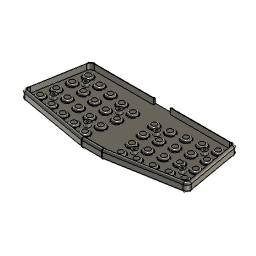
pusheenz40 low tolerance v5 (Autodesk Fusion 360 design; units mm, degrees)
Autodesk Fusion 360 part; units mm, degrees
note: some values were not read from the file. Chosen so that the rebuilt part matches the saved one: which bodies a step acts on. Set by a fixed rule: which sketch regions a step uses.
(part 1 of 2)
sketch "Sketch1" plane through (0, 0, 0) normal (0, 0, 1) x (1, 0, 0)
  line L0 (-7.5882, -2.7237) -> (-0.9058, 35.1744)
  line L1 (2.0486, 37.6534) -> (102.6819, 37.6534)
  line L2 (105.6363, 35.1744) -> (112.3188, -2.7237)
  line L3 (109.8853, -6.1991) -> (59.9186, -15.0095)
  line L4 (59.3977, -15.0551) -> (45.3329, -15.0551)
  line L5 (44.8119, -15.0095) -> (-5.1548, -6.1991)
  arc A0 (2.0486, 37.6534) -> (-0.9058, 35.1744) centre (2.0486, 34.6534) ccw
  arc A1 (105.6363, 35.1744) -> (102.6819, 37.6534) centre (102.6819, 34.6534) ccw
  arc A2 (109.8853, -6.1991) -> (112.3188, -2.7237) centre (109.3644, -3.2446) ccw
  arc A3 (59.3977, -15.0551) -> (59.9186, -15.0095) centre (59.3977, -12.0551) ccw
  arc A4 (44.8119, -15.0095) -> (45.3329, -15.0551) centre (45.3329, -12.0551) ccw
  arc A5 (-7.5882, -2.7237) -> (-5.1548, -6.1991) centre (-4.6338, -3.2446) ccw
  line L6 (-5.8506, -1.507) -> (0.3109, 33.4367)
  line L7 (3.2654, 35.9157) -> (101.4652, 35.9157)
  line L8 (104.4196, 33.4367) -> (110.5811, -1.507)
  line L9 (108.1476, -4.9823) -> (61.1353, -13.2719)
  line L10 (60.6144, -13.3174) -> (44.1162, -13.3174)
  line L11 (43.5952, -13.2719) -> (-3.4171, -4.9823)
  arc A6 (3.2654, 35.9157) -> (0.3109, 33.4367) centre (3.2654, 32.9157) ccw
  arc A7 (104.4196, 33.4367) -> (101.4652, 35.9157) centre (101.4652, 32.9157) ccw
  arc A8 (108.1476, -4.9823) -> (110.5811, -1.507) centre (107.6267, -2.0279) ccw
  arc A9 (60.6144, -13.3174) -> (61.1353, -13.2719) centre (60.6144, -10.3174) ccw
  arc A10 (43.5952, -13.2719) -> (44.1162, -13.3174) centre (44.1162, -10.3174) ccw
  arc A11 (-5.8506, -1.507) -> (-3.4171, -4.9823) centre (-2.8961, -2.0279) ccw
  line L12 (-5.2713, -1.1014) -> (0.7165, 32.8575)
  line L13 (3.6709, 35.3365) -> (101.0596, 35.3365)
  line L14 (104.014, 32.8575) -> (110.0019, -1.1014)
  line L15 (107.5684, -4.5767) -> (61.5409, -12.6926)
  line L16 (61.02, -12.7382) -> (43.7106, -12.7382)
  line L17 (43.1896, -12.6926) -> (-2.8379, -4.5767)
  arc A12 (3.6709, 35.3365) -> (0.7165, 32.8575) centre (3.6709, 32.3365) ccw
  arc A13 (104.014, 32.8575) -> (101.0596, 35.3365) centre (101.0596, 32.3365) ccw
  arc A14 (107.5684, -4.5767) -> (110.0019, -1.1014) centre (107.0475, -1.6223) ccw
  arc A15 (61.02, -12.7382) -> (61.5409, -12.6926) centre (61.02, -9.7382) ccw
  arc A16 (43.1896, -12.6926) -> (43.7106, -12.7382) centre (43.7106, -9.7382) ccw
  arc A17 (-5.2713, -1.1014) -> (-2.8379, -4.5767) centre (-2.3169, -1.6223) ccw
  arc A18 (-3.5838, -0.4343) -> (3.2191, -1.6338) centre (0, 0) ccw
  arc A19 (3.5838, 0.4343) -> (-3.2191, 1.6338) centre (0, 0) ccw
  arc A20 (-1.8473, 9.4138) -> (4.9556, 8.2143) centre (1.7365, 9.8481) ccw
  arc A21 (5.3203, 10.2824) -> (-1.4826, 11.4819) centre (1.7365, 9.8481) ccw
  arc A22 (-0.1108, 19.2619) -> (6.6921, 18.0623) centre (3.473, 19.6962) ccw
  arc A23 (7.0567, 20.1304) -> (0.2538, 21.33) centre (3.473, 19.6962) ccw
  arc A24 (1.6257, 29.11) -> (8.4286, 27.9104) centre (5.2094, 29.5442) ccw
  arc A25 (8.7932, 29.9785) -> (1.9903, 31.178) centre (5.2094, 29.5442) ccw
  arc A26 (6.2643, -2.1708) -> (13.0672, -3.3703) centre (9.8481, -1.7365) ccw
  arc A27 (13.4319, -1.3022) -> (6.629, -0.1027) centre (9.8481, -1.7365) ccw
  arc A28 (8.0008, 7.6773) -> (14.8037, 6.4778) centre (11.5846, 8.1116) ccw
  arc A29 (15.1683, 8.5459) -> (8.3654, 9.7454) centre (11.5846, 8.1116) ccw
  arc A30 (9.7373, 17.5254) -> (16.5402, 16.3259) centre (13.321, 17.9597) ccw
  arc A31 (16.9048, 18.394) -> (10.1019, 19.5935) centre (13.321, 17.9597) ccw
  arc A32 (11.4737, 27.3735) -> (18.2766, 26.1739) centre (15.0575, 27.8078) ccw
  arc A33 (18.6413, 28.242) -> (11.8384, 29.4416) centre (15.0575, 27.8078) ccw
  arc A34 (16.1124, -3.9072) -> (22.9153, -5.1068) centre (19.6962, -3.473) ccw
  arc A35 (23.2799, -3.0387) -> (16.477, -1.8391) centre (19.6962, -3.473) ccw
  arc A36 (17.8489, 5.9408) -> (24.6518, 4.7413) centre (21.4326, 6.3751) ccw
  arc A37 (25.0164, 6.8094) -> (18.2135, 8.0089) centre (21.4326, 6.3751) ccw
  arc A38 (19.5853, 15.7889) -> (26.3882, 14.5894) centre (23.1691, 16.2232) ccw
  arc A39 (26.7529, 16.6575) -> (19.95, 17.857) centre (23.1691, 16.2232) ccw
  arc A40 (21.3218, 25.637) -> (28.1247, 24.4375) centre (24.9056, 26.0713) ccw
  arc A41 (28.4894, 26.5055) -> (21.6865, 27.7051) centre (24.9056, 26.0713) ccw
  arc A42 (25.9604, -5.6437) -> (32.7634, -6.8433) centre (29.5442, -5.2094) ccw
  arc A43 (33.128, -4.7752) -> (26.3251, -3.5756) centre (29.5442, -5.2094) ccw
  arc A44 (27.6969, 4.2044) -> (34.4998, 3.0048) centre (31.2807, 4.6386) ccw
  arc A45 (34.8645, 5.0729) -> (28.0616, 6.2724) centre (31.2807, 4.6386) ccw
  arc A46 (29.4334, 14.0524) -> (36.2363, 12.8529) centre (33.0172, 14.4867) ccw
  arc A47 (36.601, 14.921) -> (29.7981, 16.1205) centre (33.0172, 14.4867) ccw
  arc A48 (31.1699, 23.9005) -> (37.9728, 22.701) centre (34.7537, 24.3348) ccw
  arc A49 (38.3375, 24.7691) -> (31.5346, 25.9686) centre (34.7537, 24.3348) ccw
  arc A50 (35.8085, -7.3802) -> (42.6114, -8.5797) centre (39.3923, -6.9459) ccw
  arc A51 (42.9761, -6.5116) -> (36.1732, -5.3121) centre (39.3923, -6.9459) ccw
  arc A52 (37.545, 2.4679) -> (44.3479, 1.2683) centre (41.1288, 2.9022) ccw
  arc A53 (44.7126, 3.3364) -> (37.9097, 4.536) centre (41.1288, 2.9022) ccw
  arc A54 (39.2815, 12.3159) -> (46.0844, 11.1164) centre (42.8653, 12.7502) ccw
  arc A55 (46.4491, 13.1845) -> (39.6462, 14.384) centre (42.8653, 12.7502) ccw
  arc A56 (41.018, 22.164) -> (47.8209, 20.9645) centre (44.6018, 22.5983) ccw
  arc A57 (48.1855, 23.0326) -> (41.3826, 24.2321) centre (44.6018, 22.5983) ccw
  arc A58 (101.5114, -1.6338) -> (108.3143, -0.4343) centre (104.7305, 0) ccw
  arc A59 (107.9497, 1.6338) -> (101.1468, 0.4343) centre (104.7305, 0) ccw
  arc A60 (99.7749, 8.2143) -> (106.5778, 9.4138) centre (102.9941, 9.8481) ccw
  arc A61 (106.2132, 11.4819) -> (99.4103, 10.2824) centre (102.9941, 9.8481) ccw
  arc A62 (98.0385, 18.0623) -> (104.8414, 19.2619) centre (101.2576, 19.6962) ccw
  arc A63 (104.4767, 21.33) -> (97.6738, 20.1304) centre (101.2576, 19.6962) ccw
  arc A64 (96.302, 27.9104) -> (103.1049, 29.11) centre (99.5211, 29.5442) ccw
  arc A65 (102.7402, 31.178) -> (95.9373, 29.9785) centre (99.5211, 29.5442) ccw
  arc A66 (91.6633, -3.3703) -> (98.4663, -2.1708) centre (94.8825, -1.7365) ccw
  arc A67 (98.1016, -0.1027) -> (91.2987, -1.3022) centre (94.8825, -1.7365) ccw
  arc A68 (89.9269, 6.4778) -> (96.7298, 7.6773) centre (93.146, 8.1116) ccw
  arc A69 (96.3651, 9.7454) -> (89.5622, 8.5459) centre (93.146, 8.1116) ccw
  arc A70 (88.1904, 16.3259) -> (94.9933, 17.5254) centre (91.4095, 17.9597) ccw
  arc A71 (94.6286, 19.5935) -> (87.8257, 18.394) centre (91.4095, 17.9597) ccw
  arc A72 (86.4539, 26.1739) -> (93.2568, 27.3735) centre (89.673, 27.8078) ccw
  arc A73 (92.8921, 29.4416) -> (86.0892, 28.242) centre (89.673, 27.8078) ccw
  arc A74 (81.8153, -5.1068) -> (88.6182, -3.9072) centre (85.0344, -3.473) ccw
  arc A75 (88.2535, -1.8391) -> (81.4506, -3.0387) centre (85.0344, -3.473) ccw
  arc A76 (80.0788, 4.7413) -> (86.8817, 5.9408) centre (83.2979, 6.3751) ccw
  arc A77 (86.517, 8.0089) -> (79.7141, 6.8094) centre (83.2979, 6.3751) ccw
  arc A78 (78.3423, 14.5894) -> (85.1452, 15.7889) centre (81.5614, 16.2232) ccw
  arc A79 (84.7806, 17.857) -> (77.9776, 16.6575) centre (81.5614, 16.2232) ccw
  arc A80 (76.6058, 24.4375) -> (83.4087, 25.637) centre (79.8249, 26.0713) ccw
  arc A81 (83.0441, 27.7051) -> (76.2412, 26.5055) centre (79.8249, 26.0713) ccw
  arc A82 (71.9672, -6.8433) -> (78.7701, -5.6437) centre (75.1863, -5.2094) ccw
  arc A83 (78.4054, -3.5756) -> (71.6025, -4.7752) centre (75.1863, -5.2094) ccw
  arc A84 (70.2307, 3.0048) -> (77.0336, 4.2044) centre (73.4498, 4.6386) ccw
  arc A85 (76.669, 6.2724) -> (69.866, 5.0729) centre (73.4498, 4.6386) ccw
  arc A86 (68.4942, 12.8529) -> (75.2971, 14.0524) centre (71.7134, 14.4867) ccw
  arc A87 (74.9325, 16.1205) -> (68.1296, 14.921) centre (71.7134, 14.4867) ccw
  arc A88 (66.7577, 22.701) -> (73.5607, 23.9005) centre (69.9769, 24.3348) ccw
  arc A89 (73.196, 25.9686) -> (66.3931, 24.7691) centre (69.9769, 24.3348) ccw
  arc A90 (62.1191, -8.5797) -> (68.922, -7.3802) centre (65.3382, -6.9459) ccw
  arc A91 (68.5574, -5.3121) -> (61.7545, -6.5116) centre (65.3382, -6.9459) ccw
  arc A92 (60.3826, 1.2683) -> (67.1855, 2.4679) centre (63.6018, 2.9022) ccw
  arc A93 (66.8209, 4.536) -> (60.018, 3.3364) centre (63.6018, 2.9022) ccw
  arc A94 (58.6462, 11.1164) -> (65.4491, 12.3159) centre (61.8653, 12.7502) ccw
  arc A95 (65.0844, 14.384) -> (58.2815, 13.1845) centre (61.8653, 12.7502) ccw
  arc A96 (56.9097, 20.9645) -> (63.7126, 22.164) centre (60.1288, 22.5983) ccw
  arc A97 (63.3479, 24.2321) -> (56.545, 23.0326) centre (60.1288, 22.5983) ccw
  line L18 (-3.5838, -0.4343) -> (-3.0862, -0.522)
  line L19 (2.7215, -1.5461) -> (3.2191, -1.6338)
  line L20 (3.5838, 0.4343) -> (3.0862, 0.522)
  line L21 (-2.7215, 1.5461) -> (-3.2191, 1.6338)
  line L22 (-1.8473, 9.4138) -> (-1.3497, 9.3261)
  line L23 (4.458, 8.302) -> (4.9556, 8.2143)
  line L24 (5.3203, 10.2824) -> (4.8226, 10.3701)
  line L25 (-0.985, 11.3941) -> (-1.4826, 11.4819)
  line L26 (-0.1108, 19.2619) -> (0.3868, 19.1741)
  line L27 (6.1945, 18.1501) -> (6.6921, 18.0623)
  line L28 (7.0567, 20.1304) -> (6.5591, 20.2182)
  line L29 (0.7515, 21.2422) -> (0.2538, 21.33)
  line L30 (1.6257, 29.11) -> (2.1233, 29.0222)
  line L31 (7.9309, 27.9982) -> (8.4286, 27.9104)
  line L32 (8.7932, 29.9785) -> (8.2956, 30.0663)
  line L33 (2.4879, 31.0903) -> (1.9903, 31.178)
  line L34 (6.2643, -2.1708) -> (6.7619, -2.2585)
  line L35 (12.5696, -3.2826) -> (13.0672, -3.3703)
  line L36 (13.4319, -1.3022) -> (12.9342, -1.2145)
  line L37 (7.1266, -0.1904) -> (6.629, -0.1027)
  line L38 (8.0008, 7.6773) -> (8.4984, 7.5896)
  line L39 (14.3061, 6.5655) -> (14.8037, 6.4778)
  line L40 (15.1683, 8.5459) -> (14.6707, 8.6336)
  line L41 (8.8631, 9.6577) -> (8.3654, 9.7454)
  line L42 (9.7373, 17.5254) -> (10.2349, 17.4376)
  line L43 (16.0425, 16.4136) -> (16.5402, 16.3259)
  line L44 (16.9048, 18.394) -> (16.4072, 18.4817)
  line L45 (10.5995, 19.5057) -> (10.1019, 19.5935)
  line L46 (11.4737, 27.3735) -> (11.9714, 27.2857)
  line L47 (17.779, 26.2617) -> (18.2766, 26.1739)
  line L48 (18.6413, 28.242) -> (18.1437, 28.3298)
  line L49 (12.336, 29.3538) -> (11.8384, 29.4416)
  line L50 (16.1124, -3.9072) -> (16.61, -3.995)
  line L51 (22.4177, -5.019) -> (22.9153, -5.1068)
  line L52 (23.2799, -3.0387) -> (22.7823, -2.9509)
  line L53 (16.9747, -1.9269) -> (16.477, -1.8391)
  line L54 (17.8489, 5.9408) -> (18.3465, 5.8531)
  line L55 (24.1541, 4.829) -> (24.6518, 4.7413)
  line L56 (25.0164, 6.8094) -> (24.5188, 6.8971)
  line L57 (18.7111, 7.9212) -> (18.2135, 8.0089)
  line L58 (19.5853, 15.7889) -> (20.083, 15.7012)
  line L59 (25.8906, 14.6771) -> (26.3882, 14.5894)
  line L60 (26.7529, 16.6575) -> (26.2553, 16.7452)
  line L61 (20.4476, 17.7693) -> (19.95, 17.857)
  line L62 (21.3218, 25.637) -> (21.8194, 25.5492)
  line L63 (27.6271, 24.5252) -> (28.1247, 24.4375)
  line L64 (28.4894, 26.5055) -> (27.9918, 26.5933)
  line L65 (22.1841, 27.6173) -> (21.6865, 27.7051)
  line L66 (25.9604, -5.6437) -> (26.4581, -5.7315)
  line L67 (32.2657, -6.7555) -> (32.7634, -6.8433)
  line L68 (33.128, -4.7752) -> (32.6304, -4.6874)
  line L69 (26.8227, -3.6634) -> (26.3251, -3.5756)
  line L70 (27.6969, 4.2044) -> (28.1946, 4.1166)
  line L71 (34.0022, 3.0926) -> (34.4998, 3.0048)
  line L72 (34.8645, 5.0729) -> (34.3669, 5.1607)
  line L73 (28.5592, 6.1847) -> (28.0616, 6.2724)
  line L74 (29.4334, 14.0524) -> (29.931, 13.9647)
  line L75 (35.7387, 12.9406) -> (36.2363, 12.8529)
  line L76 (36.601, 14.921) -> (36.1034, 15.0087)
  line L77 (30.2957, 16.0328) -> (29.7981, 16.1205)
  line L78 (31.1699, 23.9005) -> (31.6675, 23.8128)
  line L79 (37.4752, 22.7887) -> (37.9728, 22.701)
  line L80 (38.3375, 24.7691) -> (37.8398, 24.8568)
  line L81 (32.0322, 25.8809) -> (31.5346, 25.9686)
  line L82 (35.8085, -7.3802) -> (36.3061, -7.468)
  line L83 (42.1138, -8.492) -> (42.6114, -8.5797)
  line L84 (42.9761, -6.5116) -> (42.4785, -6.4239)
  line L85 (36.6708, -5.3999) -> (36.1732, -5.3121)
  line L86 (37.545, 2.4679) -> (38.0426, 2.3801)
  line L87 (43.8503, 1.3561) -> (44.3479, 1.2683)
  line L88 (44.7126, 3.3364) -> (44.215, 3.4242)
  line L89 (38.4073, 4.4482) -> (37.9097, 4.536)
  line L90 (39.2815, 12.3159) -> (39.7791, 12.2282)
  line L91 (45.5868, 11.2042) -> (46.0844, 11.1164)
  line L92 (46.4491, 13.1845) -> (45.9514, 13.2723)
  line L93 (40.1438, 14.2963) -> (39.6462, 14.384)
  line L94 (41.018, 22.164) -> (41.5156, 22.0763)
  line L95 (47.3233, 21.0522) -> (47.8209, 20.9645)
  line L96 (48.1855, 23.0326) -> (47.6879, 23.1203)
  line L97 (41.8803, 24.1444) -> (41.3826, 24.2321)
  line L98 (101.5114, -1.6338) -> (102.009, -1.5461)
  line L99 (107.8167, -0.522) -> (108.3143, -0.4343)
  line L100 (107.9497, 1.6338) -> (107.452, 1.5461)
  line L101 (101.6444, 0.522) -> (101.1468, 0.4343)
  line L102 (99.7749, 8.2143) -> (100.2726, 8.302)
  line L103 (106.0802, 9.3261) -> (106.5778, 9.4138)
  line L104 (106.2132, 11.4819) -> (105.7156, 11.3941)
  line L105 (99.9079, 10.3701) -> (99.4103, 10.2824)
  line L106 (98.0385, 18.0623) -> (98.5361, 18.1501)
  line L107 (104.3437, 19.1741) -> (104.8414, 19.2619)
  line L108 (104.4767, 21.33) -> (103.9791, 21.2422)
  line L109 (98.1714, 20.2182) -> (97.6738, 20.1304)
  line L110 (96.302, 27.9104) -> (96.7996, 27.9982)
  line L111 (102.6073, 29.0222) -> (103.1049, 29.11)
  line L112 (102.7402, 31.178) -> (102.2426, 31.0903)
  line L113 (96.4349, 30.0663) -> (95.9373, 29.9785)
  line L114 (91.6633, -3.3703) -> (92.161, -3.2826)
  line L115 (97.9686, -2.2585) -> (98.4663, -2.1708)
  line L116 (98.1016, -0.1027) -> (97.604, -0.1904)
  line L117 (91.7963, -1.2145) -> (91.2987, -1.3022)
  line L118 (89.9269, 6.4778) -> (90.4245, 6.5655)
  line L119 (96.2321, 7.5896) -> (96.7298, 7.6773)
  line L120 (96.3651, 9.7454) -> (95.8675, 9.6577)
  line L121 (90.0598, 8.6336) -> (89.5622, 8.5459)
  line L122 (88.1904, 16.3259) -> (88.688, 16.4136)
  line L123 (94.4957, 17.4376) -> (94.9933, 17.5254)
  line L124 (94.6286, 19.5935) -> (94.131, 19.5057)
  line L125 (88.3233, 18.4817) -> (87.8257, 18.394)
  line L126 (86.4539, 26.1739) -> (86.9515, 26.2617)
  line L127 (92.7592, 27.2857) -> (93.2568, 27.3735)
  line L128 (92.8921, 29.4416) -> (92.3945, 29.3538)
  line L129 (86.5869, 28.3298) -> (86.0892, 28.242)
  line L130 (81.8153, -5.1068) -> (82.3129, -5.019)
  line L131 (88.1206, -3.995) -> (88.6182, -3.9072)
  line L132 (88.2535, -1.8391) -> (87.7559, -1.9269)
  line L133 (81.9482, -2.9509) -> (81.4506, -3.0387)
  line L134 (80.0788, 4.7413) -> (80.5764, 4.829)
  line L135 (86.3841, 5.8531) -> (86.8817, 5.9408)
  line L136 (86.517, 8.0089) -> (86.0194, 7.9212)
  line L137 (80.2117, 6.8971) -> (79.7141, 6.8094)
  line L138 (78.3423, 14.5894) -> (78.8399, 14.6771)
  line L139 (84.6476, 15.7012) -> (85.1452, 15.7889)
  line L140 (84.7806, 17.857) -> (84.2829, 17.7693)
  line L141 (78.4753, 16.7452) -> (77.9776, 16.6575)
  line L142 (76.6058, 24.4375) -> (77.1034, 24.5252)
  line L143 (82.9111, 25.5492) -> (83.4087, 25.637)
  line L144 (83.0441, 27.7051) -> (82.5464, 27.6173)
  line L145 (76.7388, 26.5933) -> (76.2412, 26.5055)
  line L146 (71.9672, -6.8433) -> (72.4648, -6.7555)
  line L147 (78.2725, -5.7315) -> (78.7701, -5.6437)
  line L148 (78.4054, -3.5756) -> (77.9078, -3.6634)
  line L149 (72.1002, -4.6874) -> (71.6025, -4.7752)
  line L150 (70.2307, 3.0048) -> (70.7283, 3.0926)
  line L151 (76.536, 4.1166) -> (77.0336, 4.2044)
  line L152 (76.669, 6.2724) -> (76.1713, 6.1847)
  line L153 (70.3637, 5.1607) -> (69.866, 5.0729)
  line L154 (68.4942, 12.8529) -> (68.9919, 12.9406)
  line L155 (74.7995, 13.9647) -> (75.2971, 14.0524)
  line L156 (74.9325, 16.1205) -> (74.4349, 16.0328)
  line L157 (68.6272, 15.0087) -> (68.1296, 14.921)
  line L158 (66.7577, 22.701) -> (67.2554, 22.7887)
  line L159 (73.063, 23.8128) -> (73.5607, 23.9005)
  line L160 (73.196, 25.9686) -> (72.6984, 25.8809)
  line L161 (66.8907, 24.8568) -> (66.3931, 24.7691)
  line L162 (62.1191, -8.5797) -> (62.6167, -8.492)
  line L163 (68.4244, -7.468) -> (68.922, -7.3802)
  line L164 (68.5574, -5.3121) -> (68.0597, -5.3999)
  line L165 (62.2521, -6.4239) -> (61.7545, -6.5116)
  line L166 (60.3826, 1.2683) -> (60.8803, 1.3561)
  line L167 (66.6879, 2.3801) -> (67.1855, 2.4679)
  line L168 (66.8209, 4.536) -> (66.3233, 4.4482)
  line L169 (60.5156, 3.4242) -> (60.018, 3.3364)
  line L170 (58.6462, 11.1164) -> (59.1438, 11.2042)
  line L171 (64.9514, 12.2282) -> (65.4491, 12.3159)
  line L172 (65.0844, 14.384) -> (64.5868, 14.2963)
  line L173 (58.7791, 13.2723) -> (58.2815, 13.1845)
  line L174 (56.9097, 20.9645) -> (57.4073, 21.0522)
  line L175 (63.215, 22.0763) -> (63.7126, 22.164)
  line L176 (63.3479, 24.2321) -> (62.8503, 24.1444)
  line L177 (57.0426, 23.1203) -> (56.545, 23.0326)
  arc A98 (-3.0862, -0.522) -> (-3.0862, -0.522) centre (0, 0) ccw
  arc A99 (-1.3497, 9.3261) -> (-1.3497, 9.3261) centre (1.7365, 9.8481) ccw
  arc A100 (0.3868, 19.1741) -> (0.3868, 19.1741) centre (3.473, 19.6962) ccw
  arc A101 (2.1233, 29.0222) -> (2.1233, 29.0222) centre (5.2094, 29.5442) ccw
  arc A102 (6.7619, -2.2585) -> (6.7619, -2.2585) centre (9.8481, -1.7365) ccw
  arc A103 (8.4984, 7.5896) -> (8.4984, 7.5896) centre (11.5846, 8.1116) ccw
  arc A104 (10.2349, 17.4376) -> (10.2349, 17.4376) centre (13.321, 17.9597) ccw
  arc A105 (11.9714, 27.2857) -> (11.9714, 27.2857) centre (15.0575, 27.8078) ccw
  arc A106 (16.61, -3.995) -> (16.61, -3.995) centre (19.6962, -3.473) ccw
  arc A107 (18.3465, 5.8531) -> (18.3465, 5.8531) centre (21.4326, 6.3751) ccw
  arc A108 (20.083, 15.7012) -> (20.083, 15.7012) centre (23.1691, 16.2232) ccw
  arc A109 (21.8194, 25.5492) -> (21.8194, 25.5492) centre (24.9056, 26.0713) ccw
  arc A110 (26.4581, -5.7315) -> (26.4581, -5.7315) centre (29.5442, -5.2094) ccw
  arc A111 (28.1946, 4.1166) -> (28.1946, 4.1166) centre (31.2807, 4.6386) ccw
  arc A112 (29.931, 13.9647) -> (29.931, 13.9647) centre (33.0172, 14.4867) ccw
  arc A113 (31.6675, 23.8128) -> (31.6675, 23.8128) centre (34.7537, 24.3348) ccw
  arc A114 (36.3061, -7.468) -> (36.3061, -7.468) centre (39.3923, -6.9459) ccw
  arc A115 (38.0426, 2.3801) -> (38.0426, 2.3801) centre (41.1288, 2.9022) ccw
  arc A116 (39.7791, 12.2282) -> (39.7791, 12.2282) centre (42.8653, 12.7502) ccw
  arc A117 (41.5156, 22.0763) -> (41.5156, 22.0763) centre (44.6018, 22.5983) ccw
  arc A118 (102.009, -1.5461) -> (102.009, -1.5461) centre (104.7305, 0) ccw
  arc A119 (100.2726, 8.302) -> (100.2726, 8.302) centre (102.9941, 9.8481) ccw
  arc A120 (98.5361, 18.1501) -> (98.5361, 18.1501) centre (101.2576, 19.6962) ccw
  arc A121 (96.7996, 27.9982) -> (96.7996, 27.9982) centre (99.5211, 29.5442) ccw
  arc A122 (92.161, -3.2826) -> (92.161, -3.2826) centre (94.8825, -1.7365) ccw
  arc A123 (90.4245, 6.5655) -> (90.4245, 6.5655) centre (93.146, 8.1116) ccw
  arc A124 (88.688, 16.4136) -> (88.688, 16.4136) centre (91.4095, 17.9597) ccw
  arc A125 (86.9515, 26.2617) -> (86.9515, 26.2617) centre (89.673, 27.8078) ccw
  arc A126 (82.3129, -5.019) -> (82.3129, -5.019) centre (85.0344, -3.473) ccw
  arc A127 (80.5764, 4.829) -> (80.5764, 4.829) centre (83.2979, 6.3751) ccw
  arc A128 (78.8399, 14.6771) -> (78.8399, 14.6771) centre (81.5614, 16.2232) ccw
  arc A129 (77.1034, 24.5252) -> (77.1034, 24.5252) centre (79.8249, 26.0713) ccw
  arc A130 (72.4648, -6.7555) -> (72.4648, -6.7555) centre (75.1863, -5.2094) ccw
  arc A131 (70.7283, 3.0926) -> (70.7283, 3.0926) centre (73.4498, 4.6386) ccw
  arc A132 (68.9919, 12.9406) -> (68.9919, 12.9406) centre (71.7134, 14.4867) ccw
  arc A133 (67.2554, 22.7887) -> (67.2554, 22.7887) centre (69.9769, 24.3348) ccw
  arc A134 (62.6167, -8.492) -> (62.6167, -8.492) centre (65.3382, -6.9459) ccw
  arc A135 (60.8803, 1.3561) -> (60.8803, 1.3561) centre (63.6018, 2.9022) ccw
  arc A136 (59.1438, 11.2042) -> (59.1438, 11.2042) centre (61.8653, 12.7502) ccw
  arc A137 (57.4073, 21.0522) -> (57.4073, 21.0522) centre (60.1288, 22.5983) ccw
  circle A138 centre (5.7923, 4.0558) radius 2
  circle A139 centre (9.2652, 23.752) radius 2
  circle A140 centre (35.3365, -1.1536) radius 2
  circle A141 centre (38.8095, 18.5425) radius 2
  circle A142 centre (98.9383, 4.0558) radius 2
  circle A143 centre (95.4653, 23.752) radius 2
  circle A144 centre (69.394, -1.1536) radius 2
  circle A145 centre (65.9211, 18.5425) radius 2
  circle A146 centre (5.7923, 4.0558) radius 0.75
  circle A147 centre (9.2652, 23.752) radius 0.75
  circle A148 centre (35.3365, -1.1536) radius 0.75
  circle A149 centre (38.8095, 18.5425) radius 0.75
  circle A150 centre (98.9383, 4.0558) radius 0.75
  circle A151 centre (95.4653, 23.752) radius 0.75
  circle A152 centre (69.394, -1.1536) radius 0.75
  circle A153 centre (65.9211, 18.5425) radius 0.75
  circle A154 centre (0, 0) radius 3.13
  circle A155 centre (1.7365, 9.8481) radius 3.13
  circle A156 centre (3.473, 19.6962) radius 3.13
  circle A157 centre (5.2094, 29.5442) radius 3.13
  circle A158 centre (15.0575, 27.8078) radius 3.13
  circle A159 centre (13.321, 17.9597) radius 3.13
  circle A160 centre (11.5846, 8.1116) radius 3.13
  circle A161 centre (9.8481, -1.7365) radius 3.13
  circle A162 centre (19.6962, -3.473) radius 3.13
  circle A163 centre (21.4326, 6.3751) radius 3.13
  circle A164 centre (23.1691, 16.2232) radius 3.13
  circle A165 centre (24.9056, 26.0713) radius 3.13
  circle A166 centre (34.7537, 24.3348) radius 3.13
  circle A167 centre (33.0172, 14.4867) radius 3.13
  circle A168 centre (31.2807, 4.6386) radius 3.13
  circle A169 centre (29.5442, -5.2094) radius 3.13
  circle A170 centre (39.3923, -6.9459) radius 3.13
  circle A171 centre (41.1288, 2.9022) radius 3.13
  circle A172 centre (42.8653, 12.7502) radius 3.13
  circle A173 centre (44.6018, 22.5983) radius 3.13
  circle A174 centre (60.1288, 22.5983) radius 3.13
  circle A175 centre (61.8653, 12.7502) radius 3.13
  circle A176 centre (63.6018, 2.9022) radius 3.13
  circle A177 centre (65.3382, -6.9459) radius 3.13
  circle A178 centre (75.1863, -5.2094) radius 3.13
  circle A179 centre (73.4498, 4.6386) radius 3.13
  circle A180 centre (71.7134, 14.4867) radius 3.13
  circle A181 centre (69.9769, 24.3348) radius 3.13
  circle A182 centre (79.8249, 26.0713) radius 3.13
  circle A183 centre (81.5614, 16.2232) radius 3.13
  circle A184 centre (83.2979, 6.3751) radius 3.13
  circle A185 centre (85.0344, -3.473) radius 3.13
  circle A186 centre (94.8825, -1.7365) radius 3.13
  circle A187 centre (93.146, 8.1116) radius 3.13
  circle A188 centre (91.4095, 17.9597) radius 3.13
  circle A189 centre (89.673, 27.8078) radius 3.13
  circle A190 centre (99.5211, 29.5442) radius 3.13
  circle A191 centre (101.2576, 19.6962) radius 3.13
  circle A192 centre (102.9941, 9.8481) radius 3.13
  circle A193 centre (104.7305, 0) radius 3.13
  constraint coincident L20.end A154
  constraint concentric A21 A155
  constraint coincident L24.end A155
  constraint concentric A22 A156
  constraint coincident L28.end A156
  constraint concentric A25 A157
  constraint coincident L32.end A157
  constraint concentric A105 A158
  constraint coincident L48.end A158
  constraint concentric A31 A159
  constraint coincident L44.end A159
  constraint concentric A29 A160
  constraint coincident L40.end A160
  constraint concentric A27 A161
  constraint coincident L36.end A161
  constraint concentric A34 A162
  constraint coincident L52.end A162
  constraint coincident L56.end A163
  constraint concentric A38 A164
  constraint coincident L60.end A164
  constraint concentric A41 A165
  constraint coincident L64.end A165
  constraint coincident L80.end A166
  constraint concentric A46 A167
  constraint coincident L76.end A167
  constraint concentric A44 A168
  constraint coincident L72.end A168
  constraint coincident L68.end A169
  constraint concentric A50 A170
  constraint coincident L84.end A170
  constraint concentric A53 A171
  constraint coincident L88.end A171
  constraint coincident L92.end A172
  constraint concentric A56 A173
  constraint coincident L96.end A173
  constraint coincident L176.end A174
  constraint coincident L172.end A175
  constraint coincident L168.end A176
  constraint coincident L164.end A177
  constraint concentric A82 A178
  constraint coincident L148.end A178
  constraint concentric A84 A179
  constraint coincident L152.end A179
  constraint concentric A87 A180
  constraint coincident L156.end A180
  constraint coincident L160.end A181
  constraint coincident L144.end A182
  constraint concentric A78 A183
  constraint coincident L140.end A183
  constraint concentric A77 A184
  constraint coincident L136.end A184
  constraint concentric A75 A185
  constraint coincident L132.end A185
  constraint concentric A122 A186
  constraint coincident L116.end A186
  constraint concentric A68 A187
  constraint coincident L120.end A187
  constraint concentric A70 A188
  constraint coincident L124.end A188
  constraint coincident L128.end A189
  constraint concentric A65 A190
  constraint coincident L112.end A190
  constraint concentric A63 A191
  constraint coincident L108.end A191
  constraint concentric A60 A192
  constraint coincident L104.end A192
  constraint concentric A58 A193
  constraint coincident L99.start A193
sketch "Sketch2" plane through (0, 0, 0) normal (0, 0, 1) x (1, 0, 0)
  arc A0 (-3.4682, -0.6577) -> (3.0341, -1.8043) centre (0, 0) ccw
  arc A1 (3.4682, 0.6577) -> (-3.0341, 1.8043) centre (0, 0) ccw
  arc A2 (-1.7317, 9.1903) -> (4.7705, 8.0438) centre (1.7365, 9.8481) ccw
  arc A3 (5.2047, 10.5058) -> (-1.2976, 11.6523) centre (1.7365, 9.8481) ccw
  arc A4 (0.0048, 19.0384) -> (6.507, 17.8919) centre (3.473, 19.6962) ccw
  arc A5 (6.9411, 20.3539) -> (0.4389, 21.5004) centre (3.473, 19.6962) ccw
  arc A6 (1.7413, 28.8865) -> (8.2435, 27.74) centre (5.2094, 29.5442) ccw
  arc A7 (8.6776, 30.202) -> (2.1754, 31.3485) centre (5.2094, 29.5442) ccw
  arc A8 (6.3799, -2.3942) -> (12.8821, -3.5408) centre (9.8481, -1.7365) ccw
  arc A9 (13.3163, -1.0787) -> (6.814, 0.0678) centre (9.8481, -1.7365) ccw
  arc A10 (8.1164, 7.4538) -> (14.6186, 6.3073) centre (11.5846, 8.1116) ccw
  arc A11 (15.0527, 8.7693) -> (8.5505, 9.9159) centre (11.5846, 8.1116) ccw
  arc A12 (9.8529, 17.3019) -> (16.3551, 16.1554) centre (13.321, 17.9597) ccw
  arc A13 (16.7892, 18.6174) -> (10.287, 19.7639) centre (13.321, 17.9597) ccw
  arc A14 (11.5893, 27.15) -> (18.0916, 26.0035) centre (15.0575, 27.8078) ccw
  arc A15 (18.5257, 28.4655) -> (12.0235, 29.612) centre (15.0575, 27.8078) ccw
  arc A16 (16.228, -4.1307) -> (22.7302, -5.2772) centre (19.6962, -3.473) ccw
  arc A17 (23.1643, -2.8152) -> (16.6621, -1.6687) centre (19.6962, -3.473) ccw
  arc A18 (17.9645, 5.7174) -> (24.4667, 4.5708) centre (21.4326, 6.3751) ccw
  arc A19 (24.9008, 7.0329) -> (18.3986, 8.1794) centre (21.4326, 6.3751) ccw
  arc A20 (19.7009, 15.5654) -> (26.2032, 14.4189) centre (23.1691, 16.2232) ccw
  arc A21 (26.6373, 16.8809) -> (20.1351, 18.0275) centre (23.1691, 16.2232) ccw
  arc A22 (21.4374, 25.4135) -> (27.9397, 24.267) centre (24.9056, 26.0713) ccw
  arc A23 (28.3738, 26.729) -> (21.8715, 27.8755) centre (24.9056, 26.0713) ccw
  arc A24 (26.0761, -5.8672) -> (32.5783, -7.0137) centre (29.5442, -5.2094) ccw
  arc A25 (33.0124, -4.5517) -> (26.5102, -3.4052) centre (29.5442, -5.2094) ccw
  arc A26 (27.8125, 3.9809) -> (34.3148, 2.8344) centre (31.2807, 4.6386) ccw
  arc A27 (34.7489, 5.2964) -> (28.2467, 6.4429) centre (31.2807, 4.6386) ccw
  arc A28 (29.549, 13.829) -> (36.0513, 12.6824) centre (33.0172, 14.4867) ccw
  arc A29 (36.4854, 15.1445) -> (29.9831, 16.291) centre (33.0172, 14.4867) ccw
  arc A30 (31.2855, 23.677) -> (37.7877, 22.5305) centre (34.7537, 24.3348) ccw
  arc A31 (38.2219, 24.9925) -> (31.7196, 26.1391) centre (34.7537, 24.3348) ccw
  arc A32 (35.9241, -7.6037) -> (42.4264, -8.7502) centre (39.3923, -6.9459) ccw
  arc A33 (42.8605, -6.2882) -> (36.3583, -5.1417) centre (39.3923, -6.9459) ccw
  arc A34 (37.6606, 2.2444) -> (44.1629, 1.0979) centre (41.1288, 2.9022) ccw
  arc A35 (44.597, 3.5599) -> (38.0947, 4.7064) centre (41.1288, 2.9022) ccw
  arc A36 (39.3971, 12.0925) -> (45.8993, 10.946) centre (42.8653, 12.7502) ccw
  arc A37 (46.3335, 13.408) -> (39.8312, 14.5545) centre (42.8653, 12.7502) ccw
  arc A38 (41.1336, 21.9406) -> (47.6358, 20.794) centre (44.6018, 22.5983) ccw
  arc A39 (48.0699, 23.2561) -> (41.5677, 24.4026) centre (44.6018, 22.5983) ccw
  arc A40 (101.6965, -1.8043) -> (108.1987, -0.6577) centre (104.7305, 0) ccw
  arc A41 (107.7646, 1.8043) -> (101.2624, 0.6577) centre (104.7305, 0) ccw
  arc A42 (99.96, 8.0438) -> (106.4622, 9.1903) centre (102.9941, 9.8481) ccw
  arc A43 (106.0281, 11.6523) -> (99.5259, 10.5058) centre (102.9941, 9.8481) ccw
  arc A44 (98.2235, 17.8919) -> (104.7258, 19.0384) centre (101.2576, 19.6962) ccw
  arc A45 (104.2916, 21.5004) -> (97.7894, 20.3539) centre (101.2576, 19.6962) ccw
  arc A46 (96.487, 27.74) -> (102.9893, 28.8865) centre (99.5211, 29.5442) ccw
  arc A47 (102.5552, 31.3485) -> (96.0529, 30.202) centre (99.5211, 29.5442) ccw
  arc A48 (91.8484, -3.5408) -> (98.3506, -2.3942) centre (94.8825, -1.7365) ccw
  arc A49 (97.9165, 0.0678) -> (91.4143, -1.0787) centre (94.8825, -1.7365) ccw
  arc A50 (90.1119, 6.3073) -> (96.6142, 7.4538) centre (93.146, 8.1116) ccw
  arc A51 (96.18, 9.9159) -> (89.6778, 8.7693) centre (93.146, 8.1116) ccw
  arc A52 (88.3754, 16.1554) -> (94.8777, 17.3019) centre (91.4095, 17.9597) ccw
  arc A53 (94.4436, 19.7639) -> (87.9413, 18.6174) centre (91.4095, 17.9597) ccw
  arc A54 (86.639, 26.0035) -> (93.1412, 27.15) centre (89.673, 27.8078) ccw
  arc A55 (92.7071, 29.612) -> (86.2048, 28.4655) centre (89.673, 27.8078) ccw
  arc A56 (82.0003, -5.2772) -> (88.5026, -4.1307) centre (85.0344, -3.473) ccw
  arc A57 (88.0685, -1.6687) -> (81.5662, -2.8152) centre (85.0344, -3.473) ccw
  arc A58 (80.2639, 4.5708) -> (86.7661, 5.7174) centre (83.2979, 6.3751) ccw
  arc A59 (86.332, 8.1794) -> (79.8297, 7.0329) centre (83.2979, 6.3751) ccw
  arc A60 (78.5274, 14.4189) -> (85.0296, 15.5654) centre (81.5614, 16.2232) ccw
  arc A61 (84.5955, 18.0275) -> (78.0932, 16.8809) centre (81.5614, 16.2232) ccw
  arc A62 (76.7909, 24.267) -> (83.2931, 25.4135) centre (79.8249, 26.0713) ccw
  arc A63 (82.859, 27.8755) -> (76.3568, 26.729) centre (79.8249, 26.0713) ccw
  arc A64 (72.1523, -7.0137) -> (78.6545, -5.8672) centre (75.1863, -5.2094) ccw
  arc A65 (78.2204, -3.4052) -> (71.7181, -4.5517) centre (75.1863, -5.2094) ccw
  arc A66 (70.4158, 2.8344) -> (76.918, 3.9809) centre (73.4498, 4.6386) ccw
  arc A67 (76.4839, 6.4429) -> (69.9817, 5.2964) centre (73.4498, 4.6386) ccw
  arc A68 (68.6793, 12.6824) -> (75.1815, 13.829) centre (71.7134, 14.4867) ccw
  arc A69 (74.7474, 16.291) -> (68.2452, 15.1445) centre (71.7134, 14.4867) ccw
  arc A70 (66.9428, 22.5305) -> (73.445, 23.677) centre (69.9769, 24.3348) ccw
  arc A71 (73.0109, 26.1391) -> (66.5087, 24.9925) centre (69.9769, 24.3348) ccw
  arc A72 (62.3042, -8.7502) -> (68.8064, -7.6037) centre (65.3382, -6.9459) ccw
  arc A73 (68.3723, -5.1417) -> (61.8701, -6.2882) centre (65.3382, -6.9459) ccw
  arc A74 (60.5677, 1.0979) -> (67.0699, 2.2444) centre (63.6018, 2.9022) ccw
  arc A75 (66.6358, 4.7064) -> (60.1336, 3.5599) centre (63.6018, 2.9022) ccw
  arc A76 (58.8312, 10.946) -> (65.3335, 12.0925) centre (61.8653, 12.7502) ccw
  arc A77 (64.8993, 14.5545) -> (58.3971, 13.408) centre (61.8653, 12.7502) ccw
  arc A78 (57.0947, 20.794) -> (63.597, 21.9406) centre (60.1288, 22.5983) ccw
  arc A79 (63.1629, 24.4026) -> (56.6606, 23.2561) centre (60.1288, 22.5983) ccw
  line L0 (-3.4682, -0.6577) -> (-2.9569, -0.7479)
  line L1 (2.5228, -1.7141) -> (3.0341, -1.8043)
  line L2 (3.4682, 0.6577) -> (2.9569, 0.7479)
  line L3 (-2.5228, 1.7141) -> (-3.0341, 1.8043)
  line L4 (-1.7317, 9.1903) -> (-1.2204, 9.1002)
  line L5 (4.2592, 8.134) -> (4.7705, 8.0438)
  line L6 (5.2047, 10.5058) -> (4.6934, 10.596)
  line L7 (-0.7863, 11.5622) -> (-1.2976, 11.6523)
  line L8 (0.0048, 19.0384) -> (0.5161, 18.9482)
  line L9 (5.9957, 17.982) -> (6.507, 17.8919)
  line L10 (6.9411, 20.3539) -> (6.4298, 20.4441)
  line L11 (0.9502, 21.4103) -> (0.4389, 21.5004)
  line L12 (1.7413, 28.8865) -> (2.2526, 28.7963)
  line L13 (7.7322, 27.8301) -> (8.2435, 27.74)
  line L14 (8.6776, 30.202) -> (8.1663, 30.2921)
  line L15 (2.6867, 31.2583) -> (2.1754, 31.3485)
  line L16 (6.3799, -2.3942) -> (6.8912, -2.4844)
  line L17 (12.3708, -3.4506) -> (12.8821, -3.5408)
  line L18 (13.3163, -1.0787) -> (12.805, -0.9886)
  line L19 (7.3253, -0.0224) -> (6.814, 0.0678)
  line L20 (8.1164, 7.4538) -> (8.6277, 7.3637)
  line L21 (14.1073, 6.3975) -> (14.6186, 6.3073)
  line L22 (15.0527, 8.7693) -> (14.5414, 8.8595)
  line L23 (9.0618, 9.8257) -> (8.5505, 9.9159)
  line L24 (9.8529, 17.3019) -> (10.3642, 17.2118)
  line L25 (15.8438, 16.2456) -> (16.3551, 16.1554)
  line L26 (16.7892, 18.6174) -> (16.2779, 18.7076)
  line L27 (10.7983, 19.6738) -> (10.287, 19.7639)
  line L28 (11.5893, 27.15) -> (12.1006, 27.0598)
  line L29 (17.5803, 26.0936) -> (18.0916, 26.0035)
  line L30 (18.5257, 28.4655) -> (18.0144, 28.5557)
  line L31 (12.5348, 29.5219) -> (12.0235, 29.612)
  line L32 (16.228, -4.1307) -> (16.7393, -4.2209)
  line L33 (22.2189, -5.1871) -> (22.7302, -5.2772)
  line L34 (23.1643, -2.8152) -> (22.653, -2.7251)
  line L35 (17.1734, -1.7588) -> (16.6621, -1.6687)
  line L36 (17.9645, 5.7174) -> (18.4758, 5.6272)
  line L37 (23.9554, 4.661) -> (24.4667, 4.5708)
  line L38 (24.9008, 7.0329) -> (24.3895, 7.123)
  line L39 (18.9099, 8.0892) -> (18.3986, 8.1794)
  line L40 (19.7009, 15.5654) -> (20.2122, 15.4753)
  line L41 (25.6919, 14.5091) -> (26.2032, 14.4189)
  line L42 (26.6373, 16.8809) -> (26.126, 16.9711)
  line L43 (20.6464, 17.9373) -> (20.1351, 18.0275)
  line L44 (21.4374, 25.4135) -> (21.9487, 25.3234)
  line L45 (27.4284, 24.3572) -> (27.9397, 24.267)
  line L46 (28.3738, 26.729) -> (27.8625, 26.8192)
  line L47 (22.3828, 27.7854) -> (21.8715, 27.8755)
  line L48 (26.0761, -5.8672) -> (26.5874, -5.9574)
  line L49 (32.067, -6.9236) -> (32.5783, -7.0137)
  line L50 (33.0124, -4.5517) -> (32.5011, -4.4615)
  line L51 (27.0215, -3.4953) -> (26.5102, -3.4052)
  line L52 (27.8125, 3.9809) -> (28.3238, 3.8907)
  line L53 (33.8035, 2.9245) -> (34.3148, 2.8344)
  line L54 (34.7489, 5.2964) -> (34.2376, 5.3865)
  line L55 (28.758, 6.3527) -> (28.2467, 6.4429)
  line L56 (29.549, 13.829) -> (30.0603, 13.7388)
  line L57 (35.54, 12.7726) -> (36.0513, 12.6824)
  line L58 (36.4854, 15.1445) -> (35.9741, 15.2346)
  line L59 (30.4944, 16.2008) -> (29.9831, 16.291)
  line L60 (31.2855, 23.677) -> (31.7968, 23.5869)
  line L61 (37.2764, 22.6207) -> (37.7877, 22.5305)
  line L62 (38.2219, 24.9925) -> (37.7106, 25.0827)
  line L63 (32.2309, 26.0489) -> (31.7196, 26.1391)
  line L64 (35.9241, -7.6037) -> (36.4354, -7.6938)
  line L65 (41.9151, -8.66) -> (42.4264, -8.7502)
  line L66 (42.8605, -6.2882) -> (42.3492, -6.198)
  line L67 (36.8696, -5.2318) -> (36.3583, -5.1417)
  line L68 (37.6606, 2.2444) -> (38.1719, 2.1542)
  line L69 (43.6516, 1.188) -> (44.1629, 1.0979)
  line L70 (44.597, 3.5599) -> (44.0857, 3.6501)
  line L71 (38.606, 4.6163) -> (38.0947, 4.7064)
  line L72 (39.3971, 12.0925) -> (39.9084, 12.0023)
  line L73 (45.388, 11.0361) -> (45.8993, 10.946)
  line L74 (46.3335, 13.408) -> (45.8222, 13.4981)
  line L75 (40.3425, 14.4643) -> (39.8312, 14.5545)
  line L76 (41.1336, 21.9406) -> (41.6449, 21.8504)
  line L77 (47.1245, 20.8842) -> (47.6358, 20.794)
  line L78 (48.0699, 23.2561) -> (47.5586, 23.3462)
  line L79 (42.079, 24.3124) -> (41.5677, 24.4026)
  line L80 (101.6965, -1.8043) -> (102.2078, -1.7141)
  line L81 (107.6874, -0.7479) -> (108.1987, -0.6577)
  line L82 (107.7646, 1.8043) -> (107.2533, 1.7141)
  line L83 (101.7737, 0.7479) -> (101.2624, 0.6577)
  line L84 (99.96, 8.0438) -> (100.4713, 8.134)
  line L85 (105.9509, 9.1002) -> (106.4622, 9.1903)
  line L86 (106.0281, 11.6523) -> (105.5168, 11.5622)
  line L87 (100.0372, 10.596) -> (99.5259, 10.5058)
  line L88 (98.2235, 17.8919) -> (98.7348, 17.982)
  line L89 (104.2145, 18.9482) -> (104.7258, 19.0384)
  line L90 (104.2916, 21.5004) -> (103.7803, 21.4103)
  line L91 (98.3007, 20.4441) -> (97.7894, 20.3539)
  line L92 (96.487, 27.74) -> (96.9983, 27.8301)
  line L93 (102.478, 28.7963) -> (102.9893, 28.8865)
  line L94 (102.5552, 31.3485) -> (102.0439, 31.2583)
  line L95 (96.5642, 30.2921) -> (96.0529, 30.202)
  line L96 (91.8484, -3.5408) -> (92.3597, -3.4506)
  line L97 (97.8393, -2.4844) -> (98.3506, -2.3942)
  line L98 (97.9165, 0.0678) -> (97.4052, -0.0224)
  line L99 (91.9256, -0.9886) -> (91.4143, -1.0787)
  line L100 (90.1119, 6.3073) -> (90.6232, 6.3975)
  line L101 (96.1029, 7.3637) -> (96.6142, 7.4538)
  line L102 (96.18, 9.9159) -> (95.6687, 9.8257)
  line L103 (90.1891, 8.8595) -> (89.6778, 8.7693)
  line L104 (88.3754, 16.1554) -> (88.8867, 16.2456)
  line L105 (94.3664, 17.2118) -> (94.8777, 17.3019)
  line L106 (94.4436, 19.7639) -> (93.9323, 19.6738)
  line L107 (88.4526, 18.7076) -> (87.9413, 18.6174)
  line L108 (86.639, 26.0035) -> (87.1503, 26.0936)
  line L109 (92.6299, 27.0598) -> (93.1412, 27.15)
  line L110 (92.7071, 29.612) -> (92.1958, 29.5219)
  line L111 (86.7161, 28.5557) -> (86.2048, 28.4655)
  line L112 (82.0003, -5.2772) -> (82.5116, -5.1871)
  line L113 (87.9913, -4.2209) -> (88.5026, -4.1307)
  line L114 (88.0685, -1.6687) -> (87.5572, -1.7588)
  line L115 (82.0775, -2.7251) -> (81.5662, -2.8152)
  line L116 (80.2639, 4.5708) -> (80.7752, 4.661)
  line L117 (86.2548, 5.6272) -> (86.7661, 5.7174)
  line L118 (86.332, 8.1794) -> (85.8207, 8.0892)
  line L119 (80.341, 7.123) -> (79.8297, 7.0329)
  line L120 (78.5274, 14.4189) -> (79.0387, 14.5091)
  line L121 (84.5183, 15.4753) -> (85.0296, 15.5654)
  line L122 (84.5955, 18.0275) -> (84.0842, 17.9373)
  line L123 (78.6045, 16.9711) -> (78.0932, 16.8809)
  line L124 (76.7909, 24.267) -> (77.3022, 24.3572)
  line L125 (82.7818, 25.3234) -> (83.2931, 25.4135)
  line L126 (82.859, 27.8755) -> (82.3477, 27.7854)
  line L127 (76.8681, 26.8192) -> (76.3568, 26.729)
  line L128 (72.1523, -7.0137) -> (72.6636, -6.9236)
  line L129 (78.1432, -5.9574) -> (78.6545, -5.8672)
  line L130 (78.2204, -3.4052) -> (77.7091, -3.4953)
  line L131 (72.2294, -4.4615) -> (71.7181, -4.5517)
  line L132 (70.4158, 2.8344) -> (70.9271, 2.9245)
  line L133 (76.4067, 3.8907) -> (76.918, 3.9809)
  line L134 (76.4839, 6.4429) -> (75.9726, 6.3527)
  line L135 (70.493, 5.3865) -> (69.9817, 5.2964)
  line L136 (68.6793, 12.6824) -> (69.1906, 12.7726)
  line L137 (74.6702, 13.7388) -> (75.1815, 13.829)
  line L138 (74.7474, 16.291) -> (74.2361, 16.2008)
  line L139 (68.7565, 15.2346) -> (68.2452, 15.1445)
  line L140 (66.9428, 22.5305) -> (67.4541, 22.6207)
  line L141 (72.9337, 23.5869) -> (73.445, 23.677)
  line L142 (73.0109, 26.1391) -> (72.4996, 26.0489)
  line L143 (67.02, 25.0827) -> (66.5087, 24.9925)
  line L144 (62.3042, -8.7502) -> (62.8155, -8.66)
  line L145 (68.2951, -7.6938) -> (68.8064, -7.6037)
  line L146 (68.3723, -5.1417) -> (67.861, -5.2318)
  line L147 (62.3814, -6.198) -> (61.8701, -6.2882)
  line L148 (60.5677, 1.0979) -> (61.079, 1.188)
  line L149 (66.5586, 2.1542) -> (67.0699, 2.2444)
  line L150 (66.6358, 4.7064) -> (66.1245, 4.6163)
  line L151 (60.6449, 3.6501) -> (60.1336, 3.5599)
  line L152 (58.8312, 10.946) -> (59.3425, 11.0361)
  line L153 (64.8222, 12.0023) -> (65.3335, 12.0925)
  line L154 (64.8993, 14.5545) -> (64.388, 14.4643)
  line L155 (58.9084, 13.4981) -> (58.3971, 13.408)
  line L156 (57.0947, 20.794) -> (57.606, 20.8842)
  line L157 (63.0857, 21.8504) -> (63.597, 21.9406)
  line L158 (63.1629, 24.4026) -> (62.6516, 24.3124)
  line L159 (57.1719, 23.3462) -> (56.6606, 23.2561)
  arc A80 (-2.5228, 1.7141) -> (-2.5228, 1.7141) centre (0, 0) ccw
  arc A81 (-0.7863, 11.5622) -> (-0.7863, 11.5622) centre (1.7365, 9.8481) ccw
  arc A82 (0.9502, 21.4103) -> (0.9502, 21.4103) centre (3.473, 19.6962) ccw
  arc A83 (2.6867, 31.2583) -> (2.6867, 31.2583) centre (5.2094, 29.5442) ccw
  arc A84 (7.3253, -0.0224) -> (7.3253, -0.0224) centre (9.8481, -1.7365) ccw
  arc A85 (9.0618, 9.8257) -> (9.0618, 9.8257) centre (11.5846, 8.1116) ccw
  arc A86 (10.7983, 19.6738) -> (10.7983, 19.6738) centre (13.321, 17.9597) ccw
  arc A87 (12.5348, 29.5219) -> (12.5348, 29.5219) centre (15.0575, 27.8078) ccw
  arc A88 (17.1734, -1.7588) -> (17.1734, -1.7588) centre (19.6962, -3.473) ccw
  arc A89 (18.9099, 8.0892) -> (18.9099, 8.0892) centre (21.4326, 6.3751) ccw
  arc A90 (20.6464, 17.9373) -> (20.6464, 17.9373) centre (23.1691, 16.2232) ccw
  arc A91 (22.3828, 27.7854) -> (22.3828, 27.7854) centre (24.9056, 26.0713) ccw
  arc A92 (27.0215, -3.4953) -> (27.0215, -3.4953) centre (29.5442, -5.2094) ccw
  arc A93 (28.758, 6.3527) -> (28.758, 6.3527) centre (31.2807, 4.6386) ccw
  arc A94 (30.4944, 16.2008) -> (30.4944, 16.2008) centre (33.0172, 14.4867) ccw
  arc A95 (32.2309, 26.0489) -> (32.2309, 26.0489) centre (34.7537, 24.3348) ccw
  arc A96 (36.8696, -5.2318) -> (36.8696, -5.2318) centre (39.3923, -6.9459) ccw
  arc A97 (38.606, 4.6163) -> (38.606, 4.6163) centre (41.1288, 2.9022) ccw
  arc A98 (40.3425, 14.4643) -> (40.3425, 14.4643) centre (42.8653, 12.7502) ccw
  arc A99 (42.079, 24.3124) -> (42.079, 24.3124) centre (44.6018, 22.5983) ccw
  arc A100 (101.7737, 0.7479) -> (101.7737, 0.7479) centre (104.7305, 0) ccw
  arc A101 (100.0372, 10.596) -> (100.0372, 10.596) centre (102.9941, 9.8481) ccw
  arc A102 (98.3007, 20.4441) -> (98.3007, 20.4441) centre (101.2576, 19.6962) ccw
  arc A103 (96.5642, 30.2921) -> (96.5642, 30.2921) centre (99.5211, 29.5442) ccw
  arc A104 (91.9256, -0.9886) -> (91.9256, -0.9886) centre (94.8825, -1.7365) ccw
  arc A105 (90.1891, 8.8595) -> (90.1891, 8.8595) centre (93.146, 8.1116) ccw
  arc A106 (88.4526, 18.7076) -> (88.4526, 18.7076) centre (91.4095, 17.9597) ccw
  arc A107 (86.7161, 28.5557) -> (86.7161, 28.5557) centre (89.673, 27.8078) ccw
  arc A108 (82.0775, -2.7251) -> (82.0775, -2.7251) centre (85.0344, -3.473) ccw
  arc A109 (80.341, 7.123) -> (80.341, 7.123) centre (83.2979, 6.3751) ccw
  arc A110 (78.6045, 16.9711) -> (78.6045, 16.9711) centre (81.5614, 16.2232) ccw
  arc A111 (76.8681, 26.8192) -> (76.8681, 26.8192) centre (79.8249, 26.0713) ccw
  arc A112 (72.2294, -4.4615) -> (72.2294, -4.4615) centre (75.1863, -5.2094) ccw
  arc A113 (70.493, 5.3865) -> (70.493, 5.3865) centre (73.4498, 4.6386) ccw
  arc A114 (68.7565, 15.2346) -> (68.7565, 15.2346) centre (71.7134, 14.4867) ccw
  arc A115 (67.02, 25.0827) -> (67.02, 25.0827) centre (69.9769, 24.3348) ccw
  arc A116 (62.3814, -6.198) -> (62.3814, -6.198) centre (65.3382, -6.9459) ccw
  arc A117 (60.6449, 3.6501) -> (60.6449, 3.6501) centre (63.6018, 2.9022) ccw
  arc A118 (58.9084, 13.4981) -> (58.9084, 13.4981) centre (61.8653, 12.7502) ccw
  arc A119 (57.1719, 23.3462) -> (57.1719, 23.3462) centre (60.1288, 22.5983) ccw
  circle A120 centre (1.7365, 9.8481) radius 3.05
  circle A121 centre (3.473, 19.6962) radius 3.05
  circle A122 centre (5.2094, 29.5442) radius 3.05
  circle A123 centre (15.0575, 27.8078) radius 3.05
  circle A124 centre (24.9056, 26.0713) radius 3.05
  circle A125 centre (34.7537, 24.3348) radius 3.05
  circle A126 centre (44.6018, 22.5983) radius 3.05
  circle A127 centre (13.321, 17.9597) radius 3.05
  circle A128 centre (23.1691, 16.2232) radius 3.05
  circle A129 centre (33.0172, 14.4867) radius 3.05
  circle A130 centre (42.8653, 12.7502) radius 3.05
  circle A131 centre (11.5846, 8.1116) radius 3.05
  circle A132 centre (21.4326, 6.3751) radius 3.05
  circle A133 centre (31.2807, 4.6386) radius 3.05
  circle A134 centre (41.1288, 2.9022) radius 3.05
  circle A135 centre (9.8481, -1.7365) radius 3.05
  circle A136 centre (29.5442, -5.2094) radius 3.05
  circle A137 centre (39.3923, -6.9459) radius 3.05
  circle A138 centre (60.1288, 22.5983) radius 3.05
  circle A139 centre (69.9769, 24.3348) radius 3.05
  circle A140 centre (79.8249, 26.0713) radius 3.05
  circle A141 centre (89.673, 27.8078) radius 3.05
  circle A142 centre (99.5211, 29.5442) radius 3.05
  circle A143 centre (61.8653, 12.7502) radius 3.05
  circle A144 centre (71.7134, 14.4867) radius 3.05
  circle A145 centre (81.5614, 16.2232) radius 3.05
  circle A146 centre (91.4095, 17.9597) radius 3.05
  circle A147 centre (101.2576, 19.6962) radius 3.05
  circle A148 centre (63.6018, 2.9022) radius 3.05
  circle A149 centre (73.4498, 4.6386) radius 3.05
  circle A150 centre (83.2979, 6.3751) radius 3.05
  circle A151 centre (93.146, 8.1116) radius 3.05
  circle A152 centre (102.9941, 9.8481) radius 3.05
  circle A153 centre (65.3382, -6.9459) radius 3.05
  circle A154 centre (75.1863, -5.2094) radius 3.05
  circle A155 centre (85.0344, -3.473) radius 3.05
  circle A156 centre (94.8825, -1.7365) radius 3.05
  circle A157 centre (104.7305, 0) radius 3.05
  circle A158 centre (19.6962, -3.473) radius 3.05
  circle A159 centre (0, 0) radius 3.05
  constraint coincident L6.end A120
  constraint coincident L10.end A121
  constraint concentric A7 A122
  constraint coincident L14.end A122
  constraint concentric A15 A123
  constraint coincident L30.end A123
  constraint concentric A23 A124
  constraint coincident L46.end A124
  constraint concentric A31 A125
  constraint coincident L62.end A125
  constraint concentric A99 A126
  constraint coincident L78.end A126
  constraint coincident L26.end A127
  constraint concentric A20 A128
  constraint coincident L42.end A128
  constraint concentric A28 A129
  constraint coincident L58.end A129
  constraint concentric A37 A130
  constraint coincident L74.end A130
  constraint concentric A11 A131
  constraint coincident L22.end A131
  constraint concentric A18 A132
  constraint coincident L38.end A132
  constraint coincident L54.end A133
  constraint concentric A35 A134
  constraint coincident L70.end A134
  constraint concentric A8 A135
  constraint coincident L18.end A135
  constraint coincident L50.end A136
  constraint concentric A32 A137
  constraint coincident L66.end A137
  constraint concentric A78 A138
  constraint coincident L158.end A138
  constraint concentric A115 A139
  constraint coincident L142.end A139
  constraint coincident L126.end A140
  constraint coincident L110.end A141
  constraint concentric A46 A142
  constraint coincident L94.end A142
  constraint coincident L154.end A143
  constraint concentric A68 A144
  constraint coincident L137.start A144
  constraint concentric A110 A145
  constraint coincident L121.start A145
  constraint coincident L105.start A146
  constraint concentric A44 A147
  constraint coincident L89.start A147
  constraint concentric A75 A148
  constraint coincident L149.start A148
  constraint concentric A66 A149
  constraint coincident L133.start A149
  constraint concentric A59 A150
  constraint coincident L117.start A150
  constraint coincident L101.start A151
  constraint concentric A43 A152
  constraint coincident L85.start A152
  constraint concentric A72 A153
  constraint coincident L145.start A153
  constraint coincident L129.start A154
  constraint concentric A108 A155
  constraint coincident L113.start A155
  constraint concentric A48 A156
  constraint coincident L97.start A156
  constraint concentric A41 A157
  constraint coincident L81.start A157
  constraint concentric A16 A158
  constraint coincident L34.end A158
  constraint concentric A0 A159
  constraint coincident L2.end A159
extrude "Extrude1" add sketch "Sketch1" along normal blind 2.5 contours L6 L7 L8 L9 L10 L11 A6 A7 A8 A9 A10 A11 | L12 L13 L14 L15 L16 L17 A12 A13 A14 A15 A16 A17 | A146 | A147 | A148 | A149 | A150 | A151 | A152 | A153 makes body 1 at (69.0519, -0.4862, 1.6667) makes body 2 at (6.5413, 4.0184, 1.6667) makes body 3 at (36.0856, -1.191, 1.6667) makes body 4 at (66.2632, 19.2099, 1.6667) makes body 5 at (98.5961, 3.3884, 0.8333) makes body 6 at (8.6253, 23.3609, 1.6667) makes body 7 at (49.6051, -3.7298, 0) makes body 8 at (39.4494, 18.9336, 1.6667) makes body 9 at (95.8075, 24.4194, 1.6667)
extrude "Extrude2" add sketch "Sketch1" along normal blind 5.1 contours A138 | A139 | A140 | A141 | A142 | A143 | A144 | A145 bodies 1 2 3 4 5 6 7 8 9